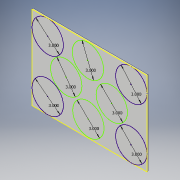
# Autodesk Inventor part: Proof of How many circles can fit in a cardboard box
Saved by Autodesk Inventor 2017 (Build 210142000, 142)
## iProperties
Created: 2020-02-10
Part Number: Proof of How many circles can fit in a cardboard box
Material: Generic
Document SubType Name: Modeling
Designer: 10042265
Density: 1 g/cm^3
Appearance: Default
Author: 10042265
Autodesk Inventor part; units mm, degrees
ref_plane "YZ Plane" through (0, 0, 0) normal (1, 0, 0) x (0, 1, 0)
ref_plane "XZ Plane" through (0, 0, 0) normal (0, 1, 0) x (-1, 0, 0)
ref_plane "XY Plane" through (0, 0, 0) normal (0, 0, 1) x (1, 0, 0)
sketch "Sketch1" plane through (0, 0, 0) normal (0, 0, 1) x (1, 0, 0)
  line L0 (0, 0) -> (279.4, 0)
  line L1 (279.4, 0) -> (279.4, 203.2)
  line L2 (279.4, 203.2) -> (0, 203.2)
  line L3 (0, 203.2) -> (0, 0)
  dimension "d0" = 279.4
  dimension "d1" = 203.2
  constraints: 8 end point, 3 perpendicular, 1 horizontal
  measures "d0" distance of L0.start L0.end
  measures "d1" distance of L0.end L1.end
extrude "Extrusion1" add sketch "Sketch1" along normal blind 3.175
sketch "Sketch2" plane through (0, 0, 3.175) normal (0, 0, 1) x (1, 0, 0)
  circle A0 centre (38.1, 38.1) radius 38.1
  line L0 (0, 203.2) -> (0, 0) projected
  line L1 (0, 0) -> (279.4, 0) projected
  circle A1 centre (241.3, 38.1) radius 38.1
  line L2 (279.4, 0) -> (279.4, 203.2) projected
  circle A2 centre (241.3, 165.1) radius 38.1
  line L3 (279.4, 203.2) -> (0, 203.2) projected
  circle A3 centre (38.1, 165.1) radius 38.1
  circle A4 centre (135.9077, 163.1391) radius 38.1
  circle A5 centre (83.1523, 101.6) radius 38.1
  circle A6 centre (193.9386, 101.6) radius 38.1
  circle A7 centre (136.9992, 39.9825) radius 38.1
  dimension "d4" = 76.2
  dimension "d5" = 76.2
  dimension "d6" = 76.2
  dimension "d7" = 76.2
  dimension "d8" = 76.2
  dimension "d9" = 76.2
  dimension "d10" = 76.2
  dimension "d11" = 76.2
  constraints: 8 centre point, 8 tangent
  measures "d4" diameter of A0
  measures "d5" diameter of A1
  measures "d6" diameter of A2
  measures "d7" diameter of A3
  measures "d8" diameter of A4
  measures "d9" diameter of A5
  measures "d10" diameter of A6
  measures "d11" diameter of A7
body "Solid1"
